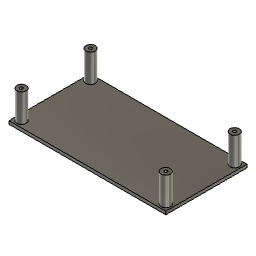
esp32-standoff (Autodesk Fusion 360 design; units mm, degrees)
Autodesk Fusion 360 part; units mm, degrees
sketch "Szkic1" plane through (0, 0, 0) normal (0, 0, 1) x (1, 0, 0)
sketch "Szkic2" plane through (0, 0, 0) normal (0, 0, 1) x (1, 0, 0)
  line L0 (-25, 25.8967) -> (25, 25.8967)
  line L1 (25, 25.8967) -> (25, -0.0036)
  line L2 (25, -0.0036) -> (-25, -0.0036)
  line L3 (-25, -0.0036) -> (-25, 25.8967)
  constraint horizontal L0
  constraint vertical L1
  constraint horizontal L2
  constraint vertical L3
cylinder "Prymityw walca1" add diameter 3 height 1 placed x (1, 0, 0) y (0, 1, 0) z (0, 0, 1) at (-23, 24, 0) makes body 1
cylinder "Prymityw walca2" add diameter 3 height 1 placed x (1, 0, 0) y (0, 1, 0) z (0, 0, 1) at (-23, 2, 0) separate body makes body 2
cylinder "Prymityw walca3" add diameter 3 height 1 placed x (1, 0, 0) y (0, 1, 0) z (0, 0, 1) at (23, 2, 0) separate body makes body 3
cylinder "Prymityw walca4" add diameter 3 height 1 placed x (1, 0, 0) y (0, 1, 0) z (0, 0, 1) at (23, 24, 0) separate body makes body 4
extrude "Wyciągnięcie proste1" add 1 faces at (-22.584, 24.1231, 1) along direction (0, 0, 1) blind 8 on bodies 1 bodies 1
extrude "Wyciągnięcie proste2" add sketch "Szkic2" against normal blind 1 bodies 1 2 3 4
extrude "Wyciągnięcie proste3" add 1 faces at (23.416, 24.1231, 1) along direction (0, 0, 1) blind 8 on bodies 1 bodies 1
extrude "Wyciągnięcie proste4" add 1 faces at (23.3292, 1.8415, 1) along direction (0, 0, 1) blind 8 on bodies 1 bodies 1
extrude "Wyciągnięcie proste5" add 1 faces at (-22.6708, 1.8415, 1) along direction (0, 0, 1) blind 8 on bodies 1 bodies 1
extrude "Wyciągnięcie proste6" add 1 faces at (-22.584, 24.1231, 9) along direction (0, 0, 1) blind 1 on bodies 1 bodies 1
extrude "Wyciągnięcie proste7" cut 1 faces at (-22.584, 24.1231, 10) along direction (0, 0, -1) blind 1 on bodies 1 bodies 1
hole "Otwór1" at (23.0189, 2.0162, 9) direction (0, 0, -1) diameter 1 depth 1 tip angle 118 bodies 1
hole "Otwór2" at (-23.0357, 1.9628, 9) direction (0, 0, -1) diameter 1 depth 1 tip angle 118 bodies 1
hole "Otwór3" at (22.9656, 24.0306, 9) direction (0, 0, -1) diameter 1 depth 1 tip angle 118 bodies 1
hole "Otwór4" at (-23, 24, 9) direction (0, 0, -1) diameter 1 depth 1 tip angle 118 bodies 1
